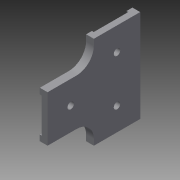
# Autodesk Inventor part: side holders
Saved by Autodesk Inventor 2015 (Build 190159000, 159)
## iProperties
Created: 2014-10-11
Part Number: side holders
Material: Generic
Document SubType Name: Modeling
Designer: jesse
Density: 1 g/cm^3
Appearance: Default
Author: jesse
Autodesk Inventor part; units mm, degrees
ref_plane "YZ Plane" through (0, 0, 0) normal (1, 0, 0) x (0, 1, 0)
ref_plane "XZ Plane" through (0, 0, 0) normal (0, 1, 0) x (-1, 0, 0)
ref_plane "XY Plane" through (0, 0, 0) normal (0, 0, 1) x (1, 0, 0)
sketch "Sketch1" plane through (0, 0, 0) normal (1, 0, 0) x (0, 1, 0)
  circle A0 centre (0, -38.1) radius 1.7907
  circle A1 centre (12.7, -12.7) radius 1.7907
  circle A2 centre (25.4, -38.1) radius 1.7907
  line L0 (-12.7, -50.8) -> (38.1, -50.8)
  line L1 (38.1, -25.4) -> (38.1, -50.8)
  line L2 (34.925, -25.4) -> (38.1, -25.4)
  arc A3 (25.4, -15.875) -> (34.925, -25.4) centre (34.925, -15.875) ccw
  line L3 (25.4, -15.875) -> (25.4, 0)
  line L4 (0, 0) -> (25.4, 0)
  line L5 (0, -15.875) -> (0, 0)
  arc A4 (-9.525, -25.4) -> (0, -15.875) centre (-9.525, -15.875) ccw
  line L6 (-9.525, -25.4) -> (-12.7, -25.4)
  line L7 (-12.7, -50.8) -> (-12.7, -25.4)
  point P0 (12.7, -50.8)
  constraints: 16 end point, 5 centre point, 4 point on circle
extrude "Extrusion1" add sketch "Sketch1" along normal blind 3.2512
sketch "Sketch2" plane through (0, 0, 0) normal (-1, 0, 0) x (0, 0, 1)
  circle A0 centre (-38.1, 25.4) radius 1.7907 projected
  circle A1 centre (-12.7, 12.7) radius 1.7907 projected
  circle A2 centre (-38.1, 0) radius 1.7907 projected
  line L0 (-50.8, -12.7) -> (-50.8, 38.1) projected
  line L1 (-25.4, -12.7) -> (-50.8, -12.7) projected
  line L2 (-25.4, -9.525) -> (-25.4, -12.7) projected
  arc A3 (-15.875, 0) -> (-25.4, -9.525) centre (-15.875, -9.525) ccw projected
  line L3 (0, 0) -> (-15.875, 0) projected
  line L4 (0, 25.4) -> (0, 0) projected
  line L5 (-15.875, 25.4) -> (0, 25.4) projected
  arc A4 (-25.4, 34.925) -> (-15.875, 25.4) centre (-15.875, 34.925) ccw projected
  line L6 (-25.4, 38.1) -> (-25.4, 34.925) projected
  line L7 (-50.8, 38.1) -> (-25.4, 38.1) projected
  line L8 (0, 25.4) -> (0, 0) projected
  line L9 (0, 22.225) -> (-28.575, 22.225)
  line L10 (0, 3.175) -> (-28.575, 3.175)
  line L11 (-28.575, 38.1) -> (-28.575, 22.225)
  line L12 (-28.575, 3.175) -> (-28.575, -12.7)
  line L13 (-25.4, -12.7) -> (-50.8, -12.7) projected
  line L14 (-47.625, 2.0848) -> (-47.625, -12.7)
  line L15 (-47.625, 2.0848) -> (-47.625, 38.1)
  line L16 (-50.8, 38.1) -> (-25.4, 38.1) projected
  line L17 (-38.1, 38.1) -> (-38.1, 48.6626) construction
  line L18 (-38.1, 52.0515) -> (-28.575, 52.0515) construction
  line L19 (-38.1, 52.0515) -> (-47.625, 52.0515) construction
  line L20 (-38.1, -12.7) -> (-38.1, -13.4551) construction
  line L21 (-38.1, -13.4551) -> (-38.1, -16.9489) construction
  line L22 (-28.575, -16.9489) -> (-38.1, -16.9489) construction
  line L23 (-38.1, -16.9489) -> (-47.625, -16.9489) construction
  line L24 (0, 12.7) -> (-6.3454, 12.7) construction
  line L25 (-3.5322, 12.7) -> (-3.5322, 22.225) construction
  line L26 (-3.5322, 12.7) -> (-3.5322, 3.175) construction
  dimension "d2" = 19.05
  dimension "d3" = 19.05
  constraints: 32 end point, 21 point on line, 4 perpendicular, 3 horizontal, 3 midpoint, 3 vertical, 2 collinear
  measures "d2" distance between parallel lines of L15 L11
  measures "d3" distance between parallel lines of L10 L9
extrude "Extrusion2" add sketch "Sketch2" along normal blind 1 contours L0 L7 L15 L14 L1 | L12 L10 L4 L3 A3 L2 L1 | L7 L6 A4 L5 L4 L9 L11
body "Solid1"
